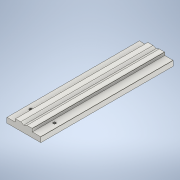
# Autodesk Inventor part: Base soporte tubos
Saved by Autodesk Inventor 2021 (Build 250183000, 183)
## iProperties
Created: 2021-04-30
Part Number: Base soporte tubos
Material: Steel AISI 1045 HV HR
Document SubType Name: Modeling
Designer: Nelson
Density: 7.85 g/cm^3
Appearance: Steel
Mass: 46341.3 g
Surface Area: 4076.9 cm^2
Volume: 5903.35 cm^3
Author: Nelson
Autodesk Inventor part; units mm, degrees
ref_plane "YZ Plane" through (0, 0, 0) normal (1, 0, 0) x (0, 1, 0)
ref_plane "XZ Plane" through (0, 0, 0) normal (0, 1, 0) x (-1, 0, 0)
ref_plane "XY Plane" through (0, 0, 0) normal (0, 0, 1) x (1, 0, 0)
sketch "Sketch1" plane through (0, 0, 0) normal (0, 0, 1) x (1, 0, 0)
  line L0 (-50, 30) -> (-50, 47.5)
  line L1 (50, 30) -> (50, 47.5)
  line L2 (-18.1144, 47.5) -> (0, 40)
  line L3 (0, 40) -> (18.1144, 47.5)
  line L4 (-100, 30) -> (-50, 30)
  line L5 (50, 30) -> (100, 30)
  line L6 (0, 40) -> (0, 46.5) construction
  line L7 (-18.1144, 47.5) -> (-50, 47.5)
  line L8 (18.1144, 47.5) -> (50, 47.5)
  line L9 (-100, 30) -> (-100, 0)
  line L10 (100, 0) -> (100, 30)
  line L11 (-100, 0) -> (0, 0)
  line L12 (0, 0) -> (100, 0)
  dimension "d90" = 17.5
  dimension "d91" = 50
  dimension "d92" = 50
  dimension "d105" = 10
  dimension "d108" = 30
  dimension "d110" = 50
  dimension "d154" = 18.1144
  constraints: 26 end point, 6 horizontal, 5 equal length, 5 vertical, 1 collinear
  measures "d90" distance of L0.start L0.end
  measures "d91" distance from line of L11.end L0
  measures "d92" distance from line of L11.end L1
  measures "d105" distance from line of L4 L2.end
  measures "d108" distance of L4.start L9.end
  measures "d110" distance of L4.start L0.start
  measures "d154" horizontal distance of L2.end L2.start
extrude "Extrusion1" add sketch "Sketch1" against normal blind 780
sketch "Sketch4" plane through (-100, 30, 0) normal (0, 1, 0) x (1, 0, 0)
  line L0 (0, 0) -> (0, 780) projected
  line L1 (50, 0) -> (0, 0) projected
  line L2 (200, 0) -> (200, 780) projected
  line L3 (200, 0) -> (150, 0) projected
  point P0 (100, 0)
  point P1 (30, 110.7)
  point P2 (170, 110.7)
  dimension "d63" = 30
  dimension "d64" = 110.7
  dimension "d65" = 30
  dimension "d109" = 110.7
  measures "d63" distance from line of L0 point (30, 110.7)
  measures "d64" distance from line of L3 point (170, 110.7)
  measures "d65" distance from line of L2 point (170, 110.7)
  measures "d109" distance from line of L1 point (30, 110.7)
hole "Hole2" at (-70, 30, -110.7) at (70, 30, -110.7) direction (0, -1, 0) diameter 15.875 depth 20 tip angle 137
thread "Thread1" size "5/8-11 UNC" class "2B" standard "ANSI Unified Screw Threads" full length
thread "Thread2" size "5/8-11 UNC" class "2B" standard "ANSI Unified Screw Threads" length 70
chamfer "Chamfer1" distance 1 angle 45 4 edges at (-50, 47.5, -390) (-100, 30, -390) (50, 47.5, -390) (100, 30, -390)
sketch "Sketch6" plane through (-100, 0, 0) normal (0, -1, 0) x (1, 0, 0)
  line L0 (190, -60) -> (190, -115.207) construction
  line L1 (190, -60) -> (167.102, -60) construction
  line L2 (167.102, -60) -> (167.102, -115.207) construction
  line L3 (100, 0) -> (100, -780) construction
  line L4 (10, -60) -> (10, -115.207) construction
  line L5 (10, -60) -> (32.898, -60) construction
  line L6 (32.898, -60) -> (32.898, -115.207) construction
  line L7 (200, -390) -> (0, -390) construction
  line L8 (0, 0) -> (0, -780) construction
  line L9 (190, -720) -> (190, -664.793) construction
  line L10 (190, -720) -> (167.102, -720) construction
  line L11 (167.102, -720) -> (167.102, -664.793) construction
  line L12 (10, -720) -> (10, -664.793) construction
  line L13 (32.898, -720) -> (32.898, -664.793) construction
  line L14 (10, -720) -> (32.898, -720) construction
  line L15 (0, 0) -> (200, 0) construction
  line L16 (200, 0) -> (200, -780) projected
  dimension "d112" = 55.207
  dimension "d113" = 22.898
  dimension "d115" = 60
  dimension "d155" = 10
  constraints: 26 end point, 21 symmetric about line, 12 coincident, 1 horizontal, 1 midpoint, 1 parallel, 1 perpendicular, 1 vertical
  measures "d112" distance of L0.start L0.end
  measures "d113" distance of L0.start L1.end
  measures "d115" distance from line of L0.start L15
  measures "d155" distance from line of L16 L0.start
hole "Hole3" at (90, 0, -60) at (90, 0, -115.207) at (67.102, 0, -60) at (67.102, 0, -115.207) at (-90, 0, -60) at (-90, 0, -115.207) at (-67.102, 0, -60) at (-67.102, 0, -115.207) at (90, 0, -720) at (90, 0, -664.793) at (67.102, 0, -720) at (67.102, 0, -664.793) at (-67.102, 0, -720) at (-67.102, 0, -664.793) at (-90, 0, -720) at (-90, 0, -664.793) direction (0, 1, 0) diameter 4.917 depth 17.1 tip angle 137 thread size "M6x1" class "6H" standard "ISO Metric profile"
sketch "Sketch8" plane through (0, 0, -780) normal (0, 0, -1) x (-1, 0, 0)
  line L0 (-100, 29) -> (-100, 0) projected
  line L1 (-100, 0) -> (100, 0) projected
  line L2 (0, 40) -> (-18.1144, 47.5) projected
  line L3 (18.1144, 47.5) -> (0, 40) projected
  point P0 (0, 0)
  point P1 (0, 20)
  dimension "d156" = 100
  dimension "d157" = 20
  measures "d156" distance from line of L0 point (0, 20)
  measures "d157" distance from line of L1 point (0, 20)
hole "Hole4" at (0, 20, -780) direction (0, 0, 1) diameter 14.376 depth 35 tip angle 137 thread size "M16x1.5" class "6H" standard "ISO Metric profile"
equation "\"d92\" = d91"
equation "\"d64\" = d109"
equation "\"d65\" = d63"
equation "\"d36\" = d34"
equation "\"d34\" = 75"
body "Solid1"
